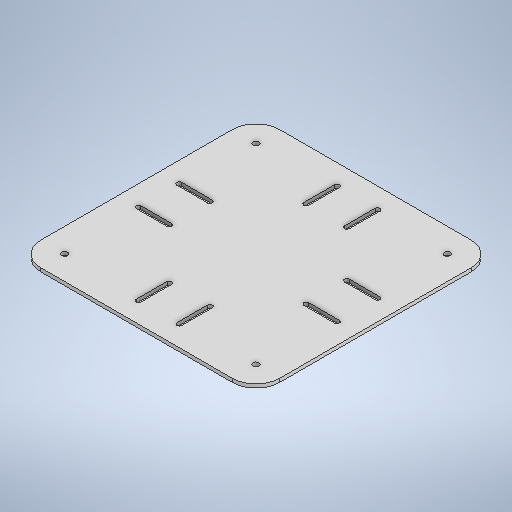
# Autodesk Inventor part: Baseprendronme
Saved by Autodesk Inventor 2025 (Build 290162010, 162A)
## iProperties
Created: 2024-11-27
Part Number: Baseprendronme
Material: Generic
Document SubType Name: Modeling
Designer: Bryan Ss
Density: 1 g/cm^3
Appearance: Default
Author: Bryan Ss
Autodesk Inventor part; units mm, degrees
ref_plane "YZ Plane" through (0, 0, 0) normal (1, 0, 0) x (0, 1, 0)
ref_plane "XZ Plane" through (0, 0, 0) normal (0, 1, 0) x (-1, 0, 0)
ref_plane "XY Plane" through (0, 0, 0) normal (0, 0, 1) x (1, 0, 0)
sketch "Sketch1" plane through (0, 0, 0) normal (0, 1, 0) x (-1, 0, 0)
  line L0 (0, 20) -> (-160, 20)
  circle A0 centre (0, -160) radius 2.5
  arc A1 (0, -180) -> (20, -160) centre (0, -160) ccw
  line L1 (0, 20) -> (-160, 20)
  arc A2 (-137.2, -66.7557) -> (-137.2, -62.7557) centre (-137.2, -64.7557) ccw
  arc A3 (-137.2, -66.7557) -> (-137.2, -62.7557) centre (-137.2, -64.7557) ccw
  line L2 (-137.2, -62.7557) -> (-163, -62.7557)
  line L3 (-137.2, -66.7557) -> (-163, -66.7557)
  arc A4 (-137.2, -100.7557) -> (-137.2, -96.7557) centre (-137.2, -98.7557) ccw
  circle A5 centre (-160, -160) radius 2.5
  circle A6 centre (-160, -160) radius 2.5
  line L4 (20, -160) -> (20, 0)
  line L5 (-180, 0) -> (-180, -160)
  line L6 (20, -160) -> (20, 0)
  line L7 (-180, 0) -> (-180, -160)
  line L8 (-160, -180) -> (0, -180)
  line L9 (-160, -180) -> (0, -180)
  arc A7 (-180, -160) -> (-160, -180) centre (-160, -160) ccw
  arc A8 (-180, -160) -> (-160, -180) centre (-160, -160) ccw
  arc A9 (-137.2, -100.7557) -> (-137.2, -96.7557) centre (-137.2, -98.7557) ccw
  arc A10 (0, -180) -> (20, -160) centre (0, -160) ccw
  circle A11 centre (0, -160) radius 2.5
  circle A12 centre (0, 0) radius 2.5
  arc A13 (20, 0) -> (0, 20) centre (0, 0) ccw
  arc A14 (20, 0) -> (0, 20) centre (0, 0) ccw
  circle A15 centre (0, 0) radius 2.5
  arc A16 (-163, -62.7557) -> (-163, -66.7557) centre (-163, -64.7557) ccw
  line L10 (-163, -96.7557) -> (-137.2, -96.7557)
  arc A17 (3, -66.7557) -> (3, -62.7557) centre (3, -64.7557) ccw
  arc A18 (3, -66.7557) -> (3, -62.7557) centre (3, -64.7557) ccw
  circle A19 centre (-160, 0) radius 2.5
  circle A20 centre (-160, 0) radius 2.5
  arc A21 (-160, 20) -> (-180, 0) centre (-160, 0) ccw
  arc A22 (-160, 20) -> (-180, 0) centre (-160, 0) ccw
  line L11 (-163, -66.7557) -> (-137.2, -66.7557)
  line L12 (-163, -100.7557) -> (-137.2, -100.7557)
  line L13 (-137.2, -100.7557) -> (-163, -100.7557)
  line L14 (-137.2, -96.7557) -> (-163, -96.7557)
  arc A23 (-163, -62.7557) -> (-163, -66.7557) centre (-163, -64.7557) ccw
  line L15 (-163, -62.7557) -> (-137.2, -62.7557)
  arc A24 (-163, -96.7557) -> (-163, -100.7557) centre (-163, -98.7557) ccw
  arc A25 (-163, -96.7557) -> (-163, -100.7557) centre (-163, -98.7557) ccw
  arc A26 (-22.8, -62.7557) -> (-22.8, -66.7557) centre (-22.8, -64.7557) ccw
  arc A27 (-22.8, -62.7557) -> (-22.8, -66.7557) centre (-22.8, -64.7557) ccw
  line L16 (-22.8, -62.7557) -> (3, -62.7557)
  line L17 (3, -62.7557) -> (-22.8, -62.7557)
  line L18 (3, -66.7557) -> (-22.8, -66.7557)
  line L19 (-22.8, -66.7557) -> (3, -66.7557)
  line L20 (-22.8, -96.7557) -> (3, -96.7557)
  line L21 (3, -96.7557) -> (-22.8, -96.7557)
  arc A28 (-22.8, -96.7557) -> (-22.8, -100.7557) centre (-22.8, -98.7557) ccw
  arc A29 (-22.8, -96.7557) -> (-22.8, -100.7557) centre (-22.8, -98.7557) ccw
  arc A30 (3, -100.7557) -> (3, -96.7557) centre (3, -98.7557) ccw
  arc A31 (3, -100.7557) -> (3, -96.7557) centre (3, -98.7557) ccw
  line L22 (3, -100.7557) -> (-22.8, -100.7557)
  line L23 (-22.8, -100.7557) -> (3, -100.7557)
  line L24 (-22.8, -66.7557) -> (3, -66.7557)
  line L25 (3, -62.7557) -> (-22.8, -62.7557)
  arc A32 (-22.8, -62.7557) -> (-22.8, -66.7557) centre (-22.8, -64.7557) ccw
  arc A33 (3, -66.7557) -> (3, -62.7557) centre (3, -64.7557) ccw
  arc A34 (20, 0) -> (0, 20) centre (0, 0) ccw
  arc A35 (20, 0) -> (0, 20) centre (0, 0) ccw
  line L26 (0, 20) -> (-160, 20)
  circle A36 centre (0, 0) radius 2.5
  circle A37 centre (0, 0) radius 2.5
  line L27 (0, 20) -> (-160, 20)
  line L28 (20, -160) -> (20, 0)
  line L29 (20, -160) -> (20, 0)
  arc A38 (0, -180) -> (20, -160) centre (0, -160) ccw
  arc A39 (0, -180) -> (20, -160) centre (0, -160) ccw
  line L30 (-66.7557, -163) -> (-66.7557, -137.2)
  line L31 (-66.7557, -137.2) -> (-66.7557, -163)
  arc A40 (-66.7557, -163) -> (-62.7557, -163) centre (-64.7557, -163) ccw
  arc A41 (-66.7557, -163) -> (-62.7557, -163) centre (-64.7557, -163) ccw
  line L32 (-96.7557, -137.2) -> (-96.7557, -163)
  line L33 (-96.7557, -163) -> (-96.7557, -137.2)
  line L34 (-100.7557, -137.2) -> (-100.7557, -163)
  line L35 (-160, -180) -> (0, -180)
  line L36 (-160, -180) -> (0, -180)
  arc A42 (-180, -160) -> (-160, -180) centre (-160, -160) ccw
  arc A43 (-100.7557, -163) -> (-96.7557, -163) centre (-98.7557, -163) ccw
  arc A44 (-180, -160) -> (-160, -180) centre (-160, -160) ccw
  arc A45 (-160, 20) -> (-180, 0) centre (-160, 0) ccw
  arc A46 (-160, 20) -> (-180, 0) centre (-160, 0) ccw
  circle A47 centre (-160, 0) radius 2.5
  circle A48 centre (-160, 0) radius 2.5
  line L37 (-180, 0) -> (-180, -160)
  line L38 (-180, 0) -> (-180, -160)
  arc A49 (-96.7557, -137.2) -> (-100.7557, -137.2) centre (-98.7557, -137.2) ccw
  circle A50 centre (-160, -160) radius 2.5
  circle A51 centre (-160, -160) radius 2.5
  arc A52 (-96.7557, -137.2) -> (-100.7557, -137.2) centre (-98.7557, -137.2) ccw
  circle A53 centre (0, -160) radius 2.5
  circle A54 centre (0, -160) radius 2.5
  line L39 (-62.7557, -163) -> (-62.7557, -137.2)
  line L40 (-62.7557, -137.2) -> (-62.7557, -163)
  arc A55 (-62.7557, -137.2) -> (-66.7557, -137.2) centre (-64.7557, -137.2) ccw
  arc A56 (-62.7557, -137.2) -> (-66.7557, -137.2) centre (-64.7557, -137.2) ccw
  line L41 (-100.7557, -163) -> (-100.7557, -137.2)
  line L42 (-96.7557, -22.8) -> (-96.7557, 3)
  line L43 (-96.7557, 3) -> (-96.7557, -22.8)
  arc A57 (-96.7557, 3) -> (-100.7557, 3) centre (-98.7557, 3) ccw
  arc A58 (-96.7557, 3) -> (-100.7557, 3) centre (-98.7557, 3) ccw
  line L44 (-100.7557, 3) -> (-100.7557, -22.8)
  arc A59 (-100.7557, -22.8) -> (-96.7557, -22.8) centre (-98.7557, -22.8) ccw
  arc A60 (-100.7557, -22.8) -> (-96.7557, -22.8) centre (-98.7557, -22.8) ccw
  line L45 (-100.7557, -22.8) -> (-100.7557, 3)
  arc A61 (-66.7557, -22.8) -> (-62.7557, -22.8) centre (-64.7557, -22.8) ccw
  line L46 (-66.7557, 3) -> (-66.7557, -22.8)
  line L47 (-66.7557, -22.8) -> (-66.7557, 3)
  arc A62 (-66.7557, -22.8) -> (-62.7557, -22.8) centre (-64.7557, -22.8) ccw
  arc A63 (-62.7557, 3) -> (-66.7557, 3) centre (-64.7557, 3) ccw
  line L48 (-62.7557, 3) -> (-62.7557, -22.8)
  line L49 (-62.7557, -22.8) -> (-62.7557, 3)
  arc A64 (-62.7557, 3) -> (-66.7557, 3) centre (-64.7557, 3) ccw
  arc A65 (-100.7557, -163) -> (-96.7557, -163) centre (-98.7557, -163) ccw
  point P0 (-22.8, -64.7557)
  point P1 (3, -64.7557)
  constraints: 100 end point, 100 point on circle, 66 centre point
extrude "Extrusion1" add sketch "Sketch1" along normal blind 3
body "Solid1"
